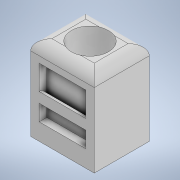
# Autodesk Inventor part: Weird_Box_Lina_Made_Me_Make_Final
Saved by Autodesk Inventor 2022 (Build 260153000, 153)
## iProperties
Created: 2023-01-25
Part Number: Weird_Box_Lina_Made_Me_Make_Final
Material: Generic
Document SubType Name: Modeling
Designer: s151859
Density: 1 g/cm^3
Appearance: Default
Author: s151859
Autodesk Inventor part; units mm, degrees
ref_plane "YZ Plane" through (0, 0, 0) normal (1, 0, 0) x (0, 1, 0)
ref_plane "XZ Plane" through (0, 0, 0) normal (0, 1, 0) x (-1, 0, 0)
ref_plane "XY Plane" through (0, 0, 0) normal (0, 0, 1) x (1, 0, 0)
sketch "Sketch1" plane through (0, 0, 0) normal (0, 1, 0) x (-1, 0, 0)
  line L0 (-9.525, -8.255) -> (9.525, -8.255)
  line L1 (9.525, -8.255) -> (9.525, 8.255)
  line L2 (9.525, 8.255) -> (-9.525, 8.255)
  line L3 (-9.525, 8.255) -> (-9.525, -8.255)
  line L4 (-9.525, -8.255) -> (9.525, 8.255) construction
  line L5 (9.525, -8.255) -> (-9.525, 8.255) construction
  point P0 (0, 0)
  dimension "d9" = 19.05
  dimension "d10" = 16.51
  constraints: 12 end point, 2 midpoint, 2 parallel, 1 horizontal, 1 perpendicular
  measures "d9" distance of L0.start L0.end
  measures "d10" distance of L2.end L0.start
extrude "Extrusion3" add sketch "Sketch1" along normal blind 25.4
sketch "actual_circle" plane through (0, 25.4, 0) normal (0, 1, 0) x (1, 0, 0)
  circle A0 centre (0, 0) radius 5.5563
  dimension "d27" = 11.1125
  constraints: 1 centre point
  measures "d27" diameter of A0
extrude "Extrusion6" cut sketch "actual_circle" against normal blind 50.8
sketch "circle" plane through (-9.525, 0, 8.255) normal (0, 0, 1) x (1, 0, 0)
  line L0 (2.54, 20.32) -> (16.51, 20.32)
  line L1 (16.51, 20.32) -> (16.51, 5.08)
  line L2 (16.51, 5.08) -> (2.54, 5.08)
  line L3 (2.54, 5.08) -> (2.54, 20.32)
  line L4 (0, 25.4) -> (19.05, 25.4) projected
  line L5 (0, 0) -> (0, 25.4) projected
  point P0 (9.525, 0)
  dimension "d32" = 13.97
  dimension "d33" = 15.24
  dimension "d34" = 5.08
  dimension "d35" = 2.54
  constraints: 8 end point, 2 parallel, 1 horizontal, 1 perpendicular
  measures "d32" distance of L0.start L0.end
  measures "d33" distance of L2.end L0.start
  measures "d34" distance between parallel lines of L4 L0
  measures "d35" distance between parallel lines of L5 L3
extrude "Extrusion7" cut sketch "circle" against normal blind 2.286
sketch "Sketch7" plane through (9.525, 0, -8.255) normal (0, 0, -1) x (-1, 0, 0)
  line L0 (2.54, 20.32) -> (16.51, 20.32)
  line L1 (16.51, 20.32) -> (16.51, 5.08)
  line L2 (16.51, 5.08) -> (2.54, 5.08)
  line L3 (2.54, 5.08) -> (2.54, 20.32)
  line L4 (0, 0) -> (0, 25.4) projected
  line L5 (0, 25.4) -> (19.05, 25.4) projected
  point P0 (9.525, 0)
  dimension "d38" = 13.97
  dimension "d39" = 15.24
  dimension "d40" = 2.54
  dimension "d41" = 5.08
  constraints: 8 end point, 2 parallel, 1 horizontal, 1 perpendicular
  measures "d38" distance of L0.start L0.end
  measures "d39" distance of L2.end L0.start
  measures "d40" distance between parallel lines of L4 L3
  measures "d41" distance between parallel lines of L5 L0
extrude "Extrusion8" cut sketch "Sketch7" against normal blind 2.286
sketch "Lock" plane through (-6.985, 5.08, -8.255) normal (1, 0, 0) x (0, 0, -1)
  line L0 (-0.762, 7.874) -> (0, 7.874)
  line L1 (0, 7.874) -> (0, 4.826)
  line L2 (0, 4.826) -> (-0.762, 4.826)
  line L3 (-0.762, 4.826) -> (-0.762, 7.874)
  line L4 (-2.286, 15.24) -> (-2.286, 0) projected
  point P0 (-8.255, -5.08)
  point P1 (0, 15.24)
  dimension "d44" = 0.762
  dimension "d45" = 3.048
  dimension "d46" = 7.366
  dimension "d47" = 1.524
  constraints: 8 end point, 2 parallel, 1 horizontal, 1 perpendicular
  measures "d44" distance of L0.start L0.end
  measures "d45" distance of L0.end L1.end
  measures "d46" distance from line of point (0, 15.24) L0
  measures "d47" distance between parallel lines of L3 L4
extrude "Extrusion9" add sketch "Lock" along normal blind 13.97
sketch "Sketch9" plane through (-6.985, 5.08, 8.255) normal (1, 0, 0) x (0, 0, -1)
  line L0 (0, 7.874) -> (0.762, 7.874)
  line L1 (0.762, 7.874) -> (0.762, 4.826)
  line L2 (0.762, 4.826) -> (0, 4.826)
  line L3 (0, 4.826) -> (0, 7.874)
  line L4 (0, 0) -> (0, 15.24) projected
  point P0 (8.255, -5.08)
  dimension "d50" = 0.762
  dimension "d51" = 3.048
  dimension "d52" = 0
  dimension "d53" = 7.366
  constraints: 8 end point, 2 parallel, 1 horizontal, 1 perpendicular
  measures "d50" distance of L0.start L0.end
  measures "d51" distance of L2.end L0.start
  measures "d52" distance between parallel lines of L4 L3
  measures "d53" distance from line of L4.end L0
extrude "Extrusion10" add sketch "Sketch9" along normal blind 13.97
fillet "Fillet1" radius 3.175 4 edges at (-9.525, 25.4, 0) (9.525, 25.4, 0) (0, 25.4, 8.255) (0, 25.4, -8.255)
body "Solid1"
